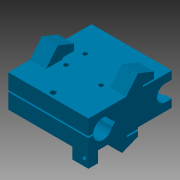
# Autodesk Inventor part: Part7
Saved by Autodesk Inventor 2015 (Build 190159000, 159)
## iProperties
Created: 2015-07-07
Part Number: Part7
Material: ABS Plastic
Document SubType Name: Modeling
Designer: hp
Density: 1.06 g/cm^3
Appearance: Sky Blue Medium
Author: hp
Autodesk Inventor part; units mm, degrees
ref_plane "YZ Plane" through (0, 0, 0) normal (1, 0, 0) x (0, 1, 0)
ref_plane "XZ Plane" through (0, 0, 0) normal (0, 1, 0) x (-1, 0, 0)
sketch "Sketch1" plane through (0, 0, 0) normal (1, 0, 0) x (0, 1, 0)
  arc A0 (5.8535, 1.7165) -> (5.8535, -1.7165) centre (0, 0) ccw
  line L0 (5.8535, 1.7165) -> (7.57, 0)
  line L1 (7.57, 0) -> (5.8535, -1.7165)
  line L2 (-9.1, 10.1) -> (43.1, 10.1)
  line L3 (43.1, -10.1) -> (-9.1, -10.1)
  line L4 (-9.1, -10.1) -> (-9.1, 10.1)
  arc A1 (39, 5.1) -> (39, -5.1) centre (39, 0) ccw
  line L5 (43.1, -10.1) -> (43.1, -5.1)
  line L6 (43.1, -5.1) -> (39, -5.1)
  line L7 (43.1, 10.1) -> (43.1, 5.1)
  line L8 (43.1, 5.1) -> (39, 5.1)
  point P0 (-9.1, 0)
  dimension "d0" = 6.1
  dimension "d1" = 7.57
  dimension "d2" = 90
  dimension "d3" = 20.2
  dimension "d4" = 52.2
  dimension "d5" = 9.1
  dimension "d6" = 5.1
  dimension "d7" = 39
  constraints: 18 end point, 4 point on circle, 3 horizontal alignment, 3 perpendicular, 3 vertical, 2 centre point, 2 tangent, 1 coincident, 1 horizontal, 1 midpoint, 1 parallel, 1 point on line
  measures "d0" radius of A0
  measures "d1" distance of L0.end point (0, 0)
  measures "d2" angle of L1 L0
  measures "d3" distance of L3.end L2.start
  measures "d4" distance of L3.start L3.end
  measures "d5" distance from line of point (0, 0) L4
  measures "d6" radius of A1
  measures "d7" distance of point (0, 0) A1.centre
extrude "Extrusion1" add sketch "Sketch1" along normal mid plane 50.2
sketch "Sketch2" plane through (-25.1, -9.1, -10.1) normal (0, -1, 0) x (1, 0, 0)
  line L0 (50.2, 0) -> (40.2, 0)
  line L1 (40.2, 0) -> (40.2, -7)
  line L2 (40.2, -7) -> (50.2, -7)
  line L3 (50.2, -7) -> (50.2, 0)
  circle A0 centre (47.2, -2) radius 1.6
  point P0 (25.1, 10.1)
  dimension "d10" = 10
  dimension "d11" = 7
  dimension "d14" = 3.2
  dimension "d15" = 3
  dimension "d16" = 5
  constraints: 8 end point, 2 parallel, 1 centre point, 1 horizontal, 1 perpendicular
  measures "d10" distance of L2.end L1.end
  measures "d11" distance of L1.end L0.end
  measures "d14" diameter of A0
  measures "d15" distance from line of L3 A0.centre
  measures "d16" distance from line of L2 A0.centre
extrude "Extrusion3" add sketch "Sketch2" against normal blind 6
ref_plane "Work Plane1" through (21.1, 0, 0) normal (1, 0, 0) x (0, 0, -1)
sketch "Sketch3" plane through (21.1, 0, 0) normal (1, 0, 0) x (0, 0, -1)
  arc A0 (-5.1, 39) -> (5.1, 39) centre (0, 39) ccw construction
  arc A1 (-6.1, 39) -> (6.1, 39) centre (0, 39) ccw
  line L0 (-6.1, 39) -> (-6.1, 43.1)
  line L1 (-5.1, 43.1) -> (-10.1, 43.1) construction
  line L2 (6.1, 39) -> (6.1, 43.1)
  line L3 (10.1, 43.1) -> (5.1, 43.1) construction
  line L4 (-6.1, 43.1) -> (6.1, 43.1)
  point P0 (0, 0)
  dimension "d20" = 6.1
  constraints: 6 end point, 2 point on circle, 2 point on line, 1 centre point, 1 coincident, 1 collinear, 1 parallel, 1 vertical
  measures "d20" radius of A1
extrude "Extrusion4" cut sketch "Sketch3" against normal blind 19.1
mirror "Mirror1" about plane through (0, 0, 0) normal (1, 0, 0) of "Extrusion4"
sketch "Sketch4" plane through (25.1, 0, 0) normal (1, 0, 0) x (0, 0, -1)
  line L0 (10.1, -3.1) -> (10.1, 43.1) projected
  line L1 (10.1, 4.5) -> (19.1, 12)
  line L2 (19.1, 12) -> (15.1, 22)
  line L3 (15.1, 22) -> (12.1, 22)
  line L4 (12.1, 22) -> (12.1, 15)
  line L5 (12.1, 15) -> (10.1, 15)
  line L6 (10.1, 15) -> (10.1, 4.5)
  line L7 (10.1, -3.1) -> (17.1, -3.1) projected
  line L8 (17.1, -9.1) -> (17.1, -3.1) projected
  point P0 (0, 0)
  dimension "d23" = 7.6
  dimension "d24" = 15.1
  dimension "d25" = 2
  dimension "d26" = 10
  dimension "d27" = 4
  dimension "d28" = 3
  dimension "d30" = 7
  constraints: 12 end point, 4 perpendicular, 2 point on line
  measures "d23" distance from line of L7 L1.start
  measures "d24" distance from line of L7 L1.end
  measures "d25" distance from line of L8 L1.end
  measures "d26" vertical distance of L1.end L2.end
  measures "d27" horizontal distance of L1.end L2.end
  measures "d28" distance of L2.end L3.end
  measures "d30" distance of L3.end L4.end
extrude "Extrusion5" add sketch "Sketch4" against normal blind 10
pattern_circular "Circular Pattern1" count 2 over 360 about axis through (0, -10, 0) along (0, 1, 0) of "Extrusion5"
sketch "Sketch5" plane through (-25.1, 0, 0) normal (-1, 0, 0) x (0, 0, 1)
  line L0 (-10.1, 43.1) -> (-10.1, -9.1) projected
  line L1 (-10.1, 14.5) -> (-19.1, 22)
  line L2 (-19.1, 22) -> (-15.1, 32)
  line L3 (-15.1, 32) -> (-12.1, 32)
  line L4 (-12.1, 32) -> (-12.1, 25)
  line L5 (-12.1, 25) -> (-10.1, 25)
  line L6 (-10.1, 25) -> (-10.1, 14.5)
  point P0 (0, 0)
  dimension "d42" = 14.5
  dimension "d43" = 7.5
  dimension "d44" = 9
  dimension "d45" = 10
  dimension "d46" = 4
  dimension "d47" = 3
  dimension "d48" = 7
  constraints: 12 end point, 3 perpendicular, 2 point on line, 1 collinear
  measures "d42" vertical distance of point (0, 0) L1.start
  measures "d43" vertical distance of L1.start L1.end
  measures "d44" horizontal distance of L1.start L1.end
  measures "d45" vertical distance of L1.end L2.end
  measures "d46" horizontal distance of L1.end L2.end
  measures "d47" distance of L2.end L3.end
  measures "d48" distance of L3.end L4.end
extrude "Extrusion6" add sketch "Sketch5" against normal blind 10
pattern_circular "Circular Pattern2" count 2 over 360 about axis through (0, -10, 0) along (0, 1, 0) of "Extrusion6"
sketch "Sketch6" plane through (-25.1, 32, -12.1) normal (0, 1, 0) x (1, 0, 0)
  line L0 (10, -2) -> (10, -1)
  line L1 (10, -2) -> (10, 7) projected
  line L2 (10, -1) -> (9, -1)
  line L3 (9, -1) -> (9, -1.9)
  line L4 (9, -1.9) -> (8, -1.9)
  line L5 (8, -1.9) -> (8, -1)
  line L6 (8, -1) -> (7, -1)
  line L7 (7, -1) -> (7, -1.9)
  line L8 (7, -1.9) -> (6, -1.9)
  line L9 (6, -1.9) -> (6, -1)
  line L10 (6, -1) -> (5, -1)
  line L11 (5, -1) -> (5, -1.9)
  line L12 (5, -1.9) -> (4, -1.9)
  line L13 (4, -1.9) -> (4, -1)
  line L14 (4, -1) -> (3, -1)
  line L15 (3, -1) -> (3, -1.9)
  line L16 (3, -1.9) -> (2, -1.9)
  line L17 (2, -1.9) -> (2, -1)
  line L18 (2, -1) -> (1, -1)
  line L19 (1, -1) -> (1, -1.9)
  line L20 (1, -1.9) -> (0, -1.9)
  line L21 (0, -1.9) -> (0, -2)
  line L22 (0, -2) -> (10, -2)
  line L23 (50.2, -24.2) -> (50.2, -23.2)
  line L24 (50.2, -23.2) -> (49.2, -23.2)
  line L25 (49.2, -23.2) -> (49.2, -24.1)
  line L26 (49.2, -24.1) -> (48.2, -24.1)
  line L27 (48.2, -24.1) -> (48.2, -23.2)
  line L28 (48.2, -23.2) -> (47.2, -23.2)
  line L29 (47.2, -23.2) -> (47.2, -24.1)
  line L30 (47.2, -24.1) -> (46.2, -24.1)
  line L31 (46.2, -24.1) -> (46.2, -23.2)
  line L32 (46.2, -23.2) -> (45.2, -23.2)
  line L33 (45.2, -23.2) -> (45.2, -24.1)
  line L34 (45.2, -24.1) -> (44.2, -24.1)
  line L35 (44.2, -24.1) -> (44.2, -23.2)
  line L36 (44.2, -23.2) -> (43.2, -23.2)
  line L37 (43.2, -23.2) -> (43.2, -24.1)
  line L38 (43.2, -24.1) -> (42.2, -24.1)
  line L39 (42.2, -24.1) -> (42.2, -23.2)
  line L40 (42.2, -23.2) -> (41.2, -23.2)
  line L41 (41.2, -23.2) -> (41.2, -24.1)
  line L42 (41.2, -24.1) -> (40.2, -24.1)
  line L43 (40.2, -27.2) -> (40.2, -24.2) projected
  line L44 (40.2, -24.1) -> (40.2, -24.2)
  line L45 (40.2, -24.2) -> (50.2, -24.2)
  point P0 (25.1, -12.1)
  dimension "d54" = 1
  dimension "d55" = 1
  dimension "d56" = 0.9
  dimension "d57" = 1
  dimension "d58" = 0.9
  dimension "d59" = 1
  dimension "d60" = 0.9
  dimension "d61" = 1
  dimension "d62" = 0.9
  dimension "d63" = 1
  dimension "d64" = 0.9
  dimension "d65" = 1
  dimension "d66" = 0.9
  dimension "d67" = 1
  dimension "d68" = 0.9
  dimension "d69" = 1
  dimension "d70" = 0.9
  dimension "d71" = 1
  dimension "d72" = 0.9
  dimension "d73" = 1
  dimension "d74" = 0.1
  dimension "d75" = 1
  dimension "d76" = 1
  dimension "d77" = 0.9
  dimension "d78" = 1
  dimension "d79" = 0.9
  dimension "d80" = 1
  dimension "d81" = 0.9
  dimension "d82" = 1
  dimension "d83" = 0.9
  dimension "d84" = 1
  dimension "d85" = 0.9
  dimension "d86" = 1
  dimension "d87" = 0.9
  dimension "d88" = 1
  dimension "d89" = 0.9
  dimension "d90" = 1
  dimension "d91" = 0.9
  dimension "d92" = 1
  dimension "d93" = 0.9
  dimension "d94" = 1
  dimension "d95" = 0.1
  constraints: 88 end point, 33 point on line, 8 vertical, 7 perpendicular, 1 horizontal
  measures "d54" distance of L0.start L0.end
  measures "d55" distance of L0.end L2.end
  measures "d56" distance of L2.end L3.end
  measures "d57" distance of L3.end L4.end
  measures "d58" distance of L4.end L5.end
  measures "d59" distance of L5.end L6.end
  measures "d60" distance of L6.end L7.end
  measures "d61" distance of L7.end L8.end
  measures "d62" distance of L8.end L9.end
  measures "d63" distance of L9.end L10.end
  measures "d64" distance of L10.end L11.end
  measures "d65" distance of L11.end L12.end
  measures "d66" distance of L12.end L13.end
  measures "d67" distance of L13.end L14.end
  measures "d68" distance of L14.end L15.end
  measures "d69" distance of L15.end L16.end
  measures "d70" distance of L16.end L17.end
  measures "d71" distance of L17.end L18.end
  measures "d72" distance of L18.end L19.end
  measures "d73" distance of L19.end L20.end
  measures "d74" distance of L20.end L21.end
  measures "d75" distance of L23.start L23.end
  measures "d76" distance of L23.end L24.end
  measures "d77" distance of L24.end L25.end
  measures "d78" distance of L25.end L26.end
  measures "d79" distance of L26.end L27.end
  measures "d80" distance of L27.end L28.end
  measures "d81" distance of L28.end L29.end
  measures "d82" distance of L29.end L30.end
  measures "d83" distance of L30.end L31.end
  measures "d84" distance of L31.end L32.end
  measures "d85" distance of L32.end L33.end
  measures "d86" distance of L33.end L34.end
  measures "d87" distance of L34.end L35.end
  measures "d88" distance of L35.end L36.end
  measures "d89" distance of L36.end L37.end
  measures "d90" distance of L37.end L38.end
  measures "d91" distance of L38.end L39.end
  measures "d92" distance of L39.end L40.end
  measures "d93" distance of L40.end L41.end
  measures "d94" distance of L41.end L42.end
  measures "d95" distance of L42.end L43.end
extrude "Extrusion7" add sketch "Sketch6" against normal blind 7
sketch "Sketch7" plane through (25.1, 22, -12.1) normal (0, 1, 0) x (1, 0, 0)
  line L0 (0, -2) -> (0, -1)
  line L1 (0, 0) -> (0, -2) projected
  line L2 (0, -1) -> (-1, -1)
  line L3 (-1, -1) -> (-1, -1.9)
  line L4 (-1, -1.9) -> (-2, -1.9)
  line L5 (-2, -1.9) -> (-2, -1)
  line L6 (-2, -1) -> (-3, -1)
  line L7 (-3, -1) -> (-3, -1.9)
  line L8 (-3, -1.9) -> (-4, -1.9)
  line L9 (-4, -1.9) -> (-4, -1)
  line L10 (-4, -1) -> (-5, -1)
  line L11 (-5, -1) -> (-5, -1.9)
  line L12 (-5, -1.9) -> (-6, -1.9)
  line L13 (-6, -1.9) -> (-6, -1)
  line L14 (-6, -1) -> (-7, -1)
  line L15 (-7, -1) -> (-7, -1.9)
  line L16 (-7, -1.9) -> (-8, -1.9)
  line L17 (-8, -1.9) -> (-8, -1)
  line L18 (-8, -1) -> (-9, -1)
  line L19 (-9, -1) -> (-9, -1.9)
  line L20 (-9, -1.9) -> (-10, -1.9)
  line L21 (-10, -1.9) -> (-10, -2)
  line L22 (-10, -2) -> (0, -2)
  line L23 (-40.2, -24.2) -> (-40.2, -23.2)
  line L24 (-40.2, -23.2) -> (-41.2, -23.2)
  line L25 (-41.2, -23.2) -> (-41.2, -24.1)
  line L26 (-50.2, -24.2) -> (-40.2, -24.2) projected
  line L27 (-41.2, -24.1) -> (-42.2, -24.1)
  line L28 (-42.2, -24.1) -> (-42.2, -23.2)
  line L29 (-42.2, -23.2) -> (-43.2, -23.2)
  line L30 (-43.2, -23.2) -> (-43.2, -24.1)
  line L31 (-43.2, -24.1) -> (-44.2, -24.1)
  line L32 (-44.2, -24.1) -> (-44.2, -23.2)
  line L33 (-44.2, -23.2) -> (-45.2, -23.2)
  line L34 (-45.2, -23.2) -> (-45.2, -24.1)
  line L35 (-45.2, -24.1) -> (-46.2, -24.1)
  line L36 (-46.2, -24.1) -> (-46.2, -23.2)
  line L37 (-46.2, -23.2) -> (-47.2, -23.2)
  line L38 (-47.2, -23.2) -> (-47.2, -24.1)
  line L39 (-47.2, -24.1) -> (-48.2, -24.1)
  line L40 (-48.2, -24.1) -> (-48.2, -23.2)
  line L41 (-48.2, -23.2) -> (-49.2, -23.2)
  line L42 (-49.2, -23.2) -> (-49.2, -24.1)
  line L43 (-49.2, -24.1) -> (-50.2, -24.1)
  line L44 (-50.2, -24.1) -> (-50.2, -24.2)
  line L45 (-50.2, -24.2) -> (-40.2, -24.2)
  point P0 (-25.1, -12.1)
  dimension "d98" = 1
  dimension "d99" = 1
  dimension "d100" = 0.9
  dimension "d101" = 1
  dimension "d102" = 0.9
  dimension "d103" = 1
  dimension "d104" = 0.9
  dimension "d105" = 1
  dimension "d106" = 0.9
  dimension "d107" = 1
  dimension "d108" = 0.9
  dimension "d109" = 1
  dimension "d110" = 0.9
  dimension "d111" = 1
  dimension "d112" = 0.9
  dimension "d113" = 1
  dimension "d114" = 0.9
  dimension "d115" = 1
  dimension "d116" = 0.9
  dimension "d117" = 1
  dimension "d118" = 0.1
  dimension "d119" = 1
  dimension "d120" = 1
  dimension "d121" = 0.9
  dimension "d123" = 1
  dimension "d124" = 0.9
  dimension "d125" = 1
  dimension "d126" = 0.9
  dimension "d127" = 1
  dimension "d128" = 0.9
  dimension "d129" = 1
  dimension "d130" = 0.9
  dimension "d131" = 1
  dimension "d132" = 0.9
  dimension "d133" = 1
  dimension "d134" = 0.9
  dimension "d135" = 1
  dimension "d136" = 0.9
  dimension "d137" = 1
  dimension "d138" = 0.9
  dimension "d139" = 1
  dimension "d140" = 0.1
  constraints: 88 end point, 21 point on line, 16 perpendicular, 9 vertical, 4 horizontal, 1 collinear, 1 midpoint
  measures "d98" distance of L0.start L0.end
  measures "d99" distance of L0.end L2.end
  measures "d100" distance of L2.end L3.end
  measures "d101" distance of L3.end L4.end
  measures "d102" distance of L4.end L5.end
  measures "d103" distance of L5.end L6.end
  measures "d104" distance of L6.end L7.end
  measures "d105" distance of L7.end L8.end
  measures "d106" distance of L8.end L9.end
  measures "d107" distance of L9.end L10.end
  measures "d108" distance of L10.end L11.end
  measures "d109" distance of L11.end L12.end
  measures "d110" distance of L12.end L13.end
  measures "d111" distance of L13.end L14.end
  measures "d112" distance of L14.end L15.end
  measures "d113" distance of L15.end L16.end
  measures "d114" distance of L16.end L17.end
  measures "d115" distance of L17.end L18.end
  measures "d116" distance of L18.end L19.end
  measures "d117" distance of L19.end L20.end
  measures "d118" distance of L20.end L21.end
  measures "d119" distance of L23.start L23.end
  measures "d120" distance of L23.end L24.end
  measures "d121" distance of L24.end L25.end
  measures "d123" distance of L25.end L27.end
  measures "d124" distance of L27.end L28.end
  measures "d125" distance of L28.end L29.end
  measures "d126" distance of L29.end L30.end
  measures "d127" distance of L30.end L31.end
  measures "d128" distance of L31.end L32.end
  measures "d129" distance of L32.end L33.end
  measures "d130" distance of L33.end L34.end
  measures "d131" distance of L34.end L35.end
  measures "d132" distance of L35.end L36.end
  measures "d133" distance of L36.end L37.end
  measures "d134" distance of L37.end L38.end
  measures "d135" distance of L38.end L39.end
  measures "d136" distance of L39.end L40.end
  measures "d137" distance of L40.end L41.end
  measures "d138" distance of L41.end L42.end
  measures "d139" distance of L42.end L43.end
  measures "d140" distance of L43.end L26.start
extrude "Extrusion8" add sketch "Sketch7" against normal blind 7
sketch "Sketch8" plane through (25.1, 0, 0) normal (1, 0, 0) x (0, 0, -1)
  line L0 (-0.5, -5.5) -> (0.5, -5.5)
  line L1 (0.5, -5.5) -> (0.5, -9.5)
  line L2 (0.5, -9.5) -> (-0.5, -9.5)
  line L3 (-0.5, -9.5) -> (-0.5, -5.5)
  point P0 (0, 0)
  point P1 (0, -5.5)
  dimension "d143" = 1
  dimension "d144" = 5.5
  dimension "d145" = 4
  constraints: 8 end point, 2 parallel, 1 horizontal, 1 midpoint, 1 perpendicular, 1 vertical alignment
  measures "d143" distance of L1.end L2.end
  measures "d144" distance from line of point (0, 0) L0
  measures "d145" distance of L0.end L1.end
extrude "Extrusion9" cut sketch "Sketch8" against normal through all
sketch "Sketch9" plane through (-25.1, 43.1, 10.1) normal (0, 0, 1) x (1, 0, 0)
  circle A0 centre (25.1, -49.1) radius 1.6
  circle A1 centre (14.1, -18.1) radius 1.3
  circle A2 centre (14.1, -30.1) radius 1.3
  circle A3 centre (36.1, -18.1) radius 1.3
  circle A4 centre (36.1, -30.1) radius 1.3
  line L0 (0, -52.2) -> (50.2, -52.2) projected
  point P0 (25.1, -43.1)
  dimension "d148" = 3.2
  dimension "d149" = 2.6
  dimension "d150" = 3.1
  dimension "d151" = 11
  dimension "d152" = 11
  dimension "d153" = 22.1
  dimension "d154" = 12
  constraints: 5 centre point, 3 equal radius, 3 vertical alignment, 2 horizontal alignment
  measures "d148" diameter of A0
  measures "d149" diameter of A1
  measures "d150" distance from line of L0 A0.centre
  measures "d151" horizontal distance of point (25.1, -43.1) A2.centre
  measures "d152" horizontal distance of point (25.1, -43.1) A4.centre
  measures "d153" distance from line of L0 A4.centre
  measures "d154" distance of A3.centre A4.centre
extrude "Extrusion10" cut sketch "Sketch9" against normal through all
equation "\"d155\" = d151"
body "Solid1"
